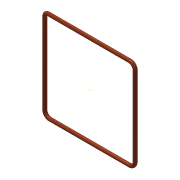
# Autodesk Inventor part: rfCoil
Saved by Autodesk Inventor 2015 (Build 190159000, 159)
## iProperties
Created: 2015-03-12
Part Number: rfCoil
Material: Generic
Document SubType Name: Modeling
Designer: jad211
Density: 1 g/cm^3
Appearance: Default
Author: jad211
Autodesk Inventor part; units mm, degrees
ref_plane "YZ Plane" through (0, 0, 0) normal (1, 0, 0) x (0, 1, 0)
ref_plane "XZ Plane" through (0, 0, 0) normal (0, 1, 0) x (-1, 0, 0)
ref_plane "XY Plane" through (0, 0, 0) normal (0, 0, 1) x (1, 0, 0)
sketch "Sketch1" plane through (0, 0, 0) normal (0, 1, 0) x (-1, 0, 0)
  line L0 (-22, 25) -> (23, 25)
  line L1 (25, 23) -> (25, -22)
  line L2 (22, -25) -> (-22, -25)
  line L3 (-25, -22) -> (-25, 22)
  line L4 (-25, 25) -> (25, -25) construction
  line L5 (25, 25) -> (-25, -25) construction
  arc A0 (25, 23) -> (23, 25) centre (23, 23) ccw
  arc A1 (22, -25) -> (25, -22) centre (22, -22) ccw
  arc A2 (-25, -22) -> (-22, -25) centre (-22, -22) ccw
  arc A3 (-22, 25) -> (-25, 22) centre (-22, 22) ccw
  point P0 (0, 0)
  dimension "d0" = 50
  dimension "d1" = 50
  dimension "d2" = 2
  dimension "d3" = 3
  constraints: 12 end point, 8 point on circle, 8 point on line, 8 tangent, 4 centre point, 2 equal radius, 2 midpoint, 2 parallel, 1 horizontal, 1 perpendicular
  measures "d0" distance of L5.start L4.end
  measures "d1" distance of L4.end L5.end
  measures "d2" radius of A0
  measures "d3" radius of A1
sketch "Sketch2" plane through (0, 0, 0) normal (0, 0, 1) x (1, 0, 0)
  point P0 (0, 0)
sketch "Sketch3" plane through (0, 0, 0) normal (0, 0, 1) x (1, 0, 0)
  circle A0 centre (25, 0) radius 0.9712
  point P0 (0, 0)
  dimension "d5" = 25
  constraints: 1 centre point
  measures "d5" distance of point (0, 0) A0.centre
sweep "Sweep1" add profiles "Sketch3" path "Sketch1"
equation "\"d1\" = d0"
equation "\"d5\" = 0.5 * d1"
body "Solid1"
